Autodesk Fusion 360 part; units mm, degrees
(part 2 of 3)
sketch "Schizzo2" plane through (0, 0, 0) normal (0, -1, 0) x (1, 0, 0)
  line L0 (-21, 0) -> (-5, 0)
  line L1 (-5, 0) -> (-5, 20)
  line L2 (-5, 20) -> (-21, 20)
  line L3 (-21, 20) -> (-21, 0)
  line L4 (-21, 10) -> (-5, 10) construction
  line L5 (-13, 20) -> (-13, 0) construction
  line L6 (-5, 8.5) -> (-21, 8.5)
  line L7 (-21, 8.5) -> (-21, 11.5)
  line L8 (-21, 11.5) -> (-5, 11.5)
  line L9 (-5, 11.5) -> (-5, 8.5)
  line L10 (-5, 8.5) -> (-21, 11.5) construction
  line L11 (-21, 8.5) -> (-5, 11.5) construction
  line L12 (-21, 20) -> (-18, 20) construction
  line L13 (-18, 20) -> (-18, 17) construction
  line L14 (-18, 17) -> (-21, 17) construction
  line L15 (-21, 17) -> (-21, 20) construction
  line L16 (-20, 15) -> (-16, 15)
  line L17 (-16, 15) -> (-16, 19)
  line L18 (-16, 19) -> (-20, 19)
  line L19 (-20, 19) -> (-20, 15)
  line L20 (-20, 15) -> (-16, 19) construction
  line L21 (-16, 15) -> (-20, 19) construction
  point P0 (-13, 10)
  point P1 (-18, 17)
  dimension "d7" = 3
  dimension "d83" = 3
  dimension "d84" = 3
  dimension "d93" = 4
  dimension "d94" = 4
  constraint midpoint L3 L4.start
  constraint midpoint L1 L4.end
  constraint midpoint L2 L5.start
  constraint midpoint L0 L5.end
  constraint horizontal L6
  constraint perpendicular L6 L7
  constraint parallel L6 L8
  constraint parallel L7 L9
  constraint coincident L10 P0
  constraint coincident L11 P0
  constraint coincident L1 L6.start
  constraint midpoint L5 P0
  constraint horizontal L12
  constraint vertical L13
  constraint horizontal L14
  constraint vertical L15
  constraint coincident L2.end L3.start
  constraint horizontal L16
  constraint perpendicular L16 L17
  constraint parallel L16 L18
  constraint parallel L17 L19
  constraint coincident L20 P1
  constraint coincident L21 P1
  constraint coincident P1 L13.end
  measures "d7" distance of L6 L8
  measures "d83" distance of L2.end L12.end
  measures "d84" distance of L2.end L14.end
  measures "d93" distance of L17.end L18.end
  measures "d94" distance of L16.end L17.end
sketch "Schizzo3" plane through (0, 140, 0) normal (0, 1, 0) x (-1, 0, 0)
  line L0 (5, 0) -> (21, 0)
  line L1 (21, 0) -> (21, 20)
  line L2 (21, 20) -> (5, 20)
  line L3 (5, 20) -> (5, 0)
  line L4 (13, 20) -> (13, 1) construction
  line L5 (5, 10) -> (21, 10) construction
  line L6 (21, 8.5) -> (5, 8.5)
  line L7 (5, 8.5) -> (5, 11.5)
  line L8 (5, 11.5) -> (21, 11.5)
  line L9 (21, 11.5) -> (21, 8.5)
  line L10 (21, 8.5) -> (5, 11.5) construction
  line L11 (5, 8.5) -> (21, 11.5) construction
  line L12 (5, 0) -> (8, 0) construction
  line L13 (8, 0) -> (8, 3) construction
  line L14 (8, 3) -> (5, 3) construction
  line L15 (5, 3) -> (5, 0) construction
  line L16 (10, 1) -> (6, 1)
  line L17 (6, 1) -> (6, 5)
  line L18 (6, 5) -> (10, 5)
  line L19 (10, 5) -> (10, 1)
  line L20 (10, 1) -> (6, 5) construction
  line L21 (6, 1) -> (10, 5) construction
  point P0 (13, 10)
  point P1 (8, 3)
  point P2 (17, 16)
  dimension "d8" = 3
  dimension "d87" = 3
  dimension "d88" = 3
  dimension "d89" = 4
  dimension "d90" = 4
  constraint midpoint L2 L4.start
  constraint perpendicular L0 L4
  constraint midpoint L3 L5.start
  constraint midpoint L1 L5.end
  constraint horizontal L6
  constraint perpendicular L6 L7
  constraint parallel L6 L8
  constraint parallel L7 L9
  constraint coincident L10 P0
  constraint coincident L11 P0
  constraint coincident L1 L6.start
  constraint midpoint L5 P0
  constraint horizontal L12
  constraint vertical L13
  constraint horizontal L14
  constraint vertical L15
  constraint coincident L0.start L3.end
  constraint horizontal L16
  constraint perpendicular L16 L17
  constraint parallel L16 L18
  constraint parallel L17 L19
  constraint coincident L20 P1
  constraint coincident L21 P1
  constraint coincident P1 L13.end
  measures "d8" distance of L6 L8
  measures "d87" distance of L0.start L12.end
  measures "d88" distance of L0.start L14.end
  measures "d89" distance of L17.end L18.end
  measures "d90" distance of L16.end L17.end
extrude "Estrusione28" cut sketch "Schizzo2" against normal blind 1 contours L16 L17 L18 L19 bodies 1
extrude "Estrusione29" cut sketch "Schizzo3" against normal blind 1 contours L16 L17 L18 L19 bodies 1
ref_plane "Piano di lavoro2" through (-8, 140, 0) normal (-0.997459, 0.071247, 0) x (-0.071247, -0.997459, 0)
sketch "Schizzo8" plane through (-17.9086, 1.2792, 0) normal (-0.997459, 0.071247, 0) x (-0.071247, -0.997459, 0)
  line L0 (1, 16) -> (-139.3, 4)
pipe "Tubo1" cut square section size 4 path "Schizzo8" along L0 bodies 1
sketch "Schizzo11" plane through (-5, 0, 0) normal (1, 0, 0) x (0, 1, 0)
  line L0 (0, 0) -> (140, 0)
  line L1 (140, 0) -> (140, 20)
  line L2 (140, 20) -> (0, 20)
  line L3 (0, 20) -> (0, 0)
  line L4 (140, 3) -> (123.5, 3) construction
  line L5 (131.75, 3) -> (131.75, 0) construction
  line L6 (123.5, 5) -> (140, 5)
  line L7 (140, 5) -> (140, 1)
  line L8 (140, 1) -> (123.5, 1)
  line L9 (123.5, 1) -> (123.5, 5)
  line L10 (123.5, 5) -> (140, 1) construction
  line L11 (140, 5) -> (123.5, 1) construction
  line L12 (0, 0) -> (140, 0)
  point P0 (131.75, 3)
  point P1 (140, 3)
  dimension "d129" = 16.5
  dimension "d132" = 4
  constraint coincident L1 P1
  constraint perpendicular L1 L4
  constraint midpoint L4 P0
  constraint coincident L0 L5.end
  constraint perpendicular L0 L5
  constraint horizontal L6
  constraint perpendicular L6 L7
  constraint parallel L6 L8
  constraint parallel L7 L9
  constraint coincident L10 P0
  constraint coincident L11 P0
  constraint coincident P0 L5.start
  constraint coincident P1 L7
  constraint coincident P1 L4.start
  measures "d129" distance of P1 L4.end
  measures "d132" distance of L6 L8
extrude "Estrusione37" cut sketch "Schizzo11" against normal blind 5 contours L1 L6 L7 L8 L9 bodies 1
sketch "Schizzo12" plane through (-21, 0, 0) normal (-1, 0, 0) x (0, -1, 0)
  line L0 (-140, 0) -> (0, 0)
  line L1 (0, 0) -> (0, 20)
  line L2 (0, 20) -> (-140, 20)
  line L3 (-140, 20) -> (-140, 0)
  line L4 (0, 17) -> (-16.5, 17) construction
  line L5 (-8.25, 17) -> (-8.25, 20) construction
  line L6 (0, 15) -> (-16.5, 15)
  line L7 (-16.5, 15) -> (-16.5, 19)
  line L8 (-16.5, 19) -> (0, 19)
  line L9 (0, 19) -> (0, 15)
  line L10 (0, 15) -> (-16.5, 19) construction
  line L11 (-16.5, 15) -> (0, 19) construction
  point P0 (0, 17)
  point P1 (-8.25, 17)
  dimension "d135" = 16.5
  dimension "d136" = 4
  constraint coincident L1 P0
  constraint perpendicular L1 L4
  constraint coincident P0 L4.start
  constraint midpoint L4 P1
  constraint coincident L2 L5.end
  constraint perpendicular L2 L5
  constraint horizontal L6
  constraint perpendicular L6 L7
  constraint parallel L6 L8
  constraint parallel L7 L9
  constraint coincident L10 P1
  constraint coincident L11 P1
  constraint coincident P1 L5.start
  constraint collinear L1 L9
  measures "d135" distance of P0 L4.end
  measures "d136" distance of L6 L8
extrude "Estrusione38" cut sketch "Schizzo12" against normal blind 5 contours L1 L6 L7 L8 L9 bodies 1
extrude "Estrusione2" cut sketch "Schizzo3" against normal blind 16.5 contours L1 L3 L6 L7 L8 L9 bodies 1
extrude "Estrusione3" cut sketch "Schizzo2" against normal blind 16.5 contours L1 L3 L6 L7 L8 L9 bodies 1
extrude "Estrusione4" cut sketch "Schizzo1" along normal blind 20 contours L0 L3 A0 L118 | L0 L1 A0 L118 | L3 A0 L118 L119 | L1 A0 L117 L118 | L3 A2 L122 L123 | L1 A2 L122 L125 | L2 L3 A2 L122 | L1 L2 A2 L122 bodies 1
extrude "Estrusione26" cut sketch "Schizzo1" along normal blind 1 contours L4 A1 A11 | L4 A1 A11 | L4 A3 A12 | L4 A3 A12 bodies 1
extrude "Estrusione120" cut sketch "Schizzo1" along normal blind 0.5 contours A0 A1 L116 L118 | L3 A0 L116 L119 picked at (-19.6721, 8.4598) bodies 1
sketch "Schizzo6" plane through (0, 0, 20) normal (0, 0, 1) x (-1, 0, 0)
  arc A0 (21, -8) -> (5, -8) centre (13, -8) ccw
  line L0 (5, -8) -> (5, -132)
  arc A1 (5, -132) -> (21, -132) centre (13, -132) ccw
  line L1 (21, -132) -> (21, -8)
  circle A2 centre (13, -132) radius 2
  circle A3 centre (13, -8) radius 2
  line L2 (13, -132) -> (13, -8) construction
  circle A4 centre (13, -132) radius 4
  line L3 (21, -70) -> (5, -70) construction
  circle A5 centre (13, -8) radius 4
  line L4 (5, -128) -> (21, -128)
  line L5 (21, -128) -> (21, -136)
  line L6 (21, -136) -> (5, -136)
  line L7 (5, -136) -> (5, -128)
  line L8 (5, -128) -> (21, -136) construction
  line L9 (21, -128) -> (5, -136) construction
  point P0 (13, -132)
  dimension "d78" = 8
  constraint coincident P0 A1.centre
  constraint coincident A0.centre A3.centre
  constraint midpoint L1 L3.start
  constraint midpoint L0 L3.end
  constraint symmetric A4 L3 A5
  constraint horizontal L4
  constraint perpendicular L4 L5
  constraint parallel L4 L6
  constraint parallel L5 L7
  constraint coincident L8 P0
  constraint coincident L9 P0
  constraint tangent A4 L6
  constraint collinear L1 L5
  measures "d78" diameter of A4
extrude "Estrusione27" cut sketch "Schizzo6" against normal blind 1 contours A4 | A5 bodies 1
extrude "Estrusione121" cut sketch "Schizzo6" against normal blind 0.5 contours L0 A1 A4 L4 L6 L7 bodies 1
extrude "Estrusione19" add sketch "Schizzo1" along normal blind 28 separate body contours L7 L11 A5 | L7 L11 A7 makes body 2
extrude "Estrusione18" add sketch "Schizzo1" along normal blind 4 contours L10 A4 A8 | L10 A4 A8 | L9 L10 L11 A4 | L10 A8 L16 | L10 A8 L16 | L7 L10 A4 A5 | L9 L10 L11 A6 | L10 L13 L14 L15 L16 A9 | L10 L12 L13 L16 L17 A9 | A8 L15 | A8 L17 | L7 L11 A5 | L10 A6 L18 L19 L22 L23 | L7 L11 A7 | L7 L10 A6 A7 | L10 A8 L13 | L10 A8 L13 | L10 A9 | L10 A9 | A8 L14 | A8 L12 | L10 A6 L19 L20 L21 L22 | L10 L19 L20 L21 L22 A10 | L10 L18 L19 L22 L23 A10 | L10 A10 | L10 A10 bodies 2
extrude "Estrusione20" cut sketch "Schizzo1" along normal blind 4 contours L10 A9 | L10 A9 | L10 A10 | L10 A10 bodies 2
extrude "Estrusione21" cut sketch "Schizzo1" along normal blind 2 contours L10 L13 L14 L15 L16 A9 | L10 L12 L13 L16 L17 A9 | L10 L19 L20 L21 L22 A10 | L10 L18 L19 L22 L23 A10 bodies 2
extrude "Estrusione22" add 1 faces at (28.834, 17.1558, 4) along direction (0, 0, 1) blind 3 from surface at 8.5 on bodies 2 bodies 2
extrude "Estrusione23" add 1 faces at (28.834, 17.1558, 15.5) along direction (0, 0, 1) blind 4 from surface at 8.5 on bodies 2 bodies 2
sketch "Schizzo5" plane through (0, 0, 28) normal (0, 0, 1) x (-1, 0, 0)
  circle A0 centre (-34.1674, -25.6558) radius 1.6
  circle A1 centre (-34.1674, -8.6558) radius 1.6
  line L0 (-42.1674, -8.6558) -> (-42.1674, -25.6558)
  arc A2 (-42.1674, -25.6558) -> (-26.1674, -25.6558) centre (-34.1674, -25.6558) ccw
  line L1 (-26.1674, -25.6558) -> (-26.1674, -8.6558)
  arc A3 (-26.1674, -8.6558) -> (-42.1674, -8.6558) centre (-34.1674, -8.6558) ccw
  line L2 (-34.1674, -8.6558) -> (-34.1674, -25.6558) construction
  circle A4 centre (-34.1674, -8.6558) radius 3
  circle A5 centre (-34.1674, -25.6558) radius 3
  circle A6 centre (-34.1674, -8.6558) radius 4
  circle A7 centre (-34.1674, -25.6558) radius 4
  dimension "d67" = 6
  dimension "d68" = 6
  dimension "d69" = 8
  dimension "d70" = 8
  constraint coincident A1.centre A3.centre
  constraint coincident A0.centre A2.centre
  constraint concentric A4 A6
  measures "d67" diameter of A4
  measures "d68" diameter of A5
  measures "d69" diameter of A6
  measures "d70" diameter of A7
extrude "Estrusione25" add sketch "Schizzo5" against normal blind 5 contours A4 | A5 | A6 | A7 bodies 2
extrude "Estrusione24" cut sketch "Schizzo5" against normal blind 3.2 contours A4 | A5 bodies 2
extrude "Estrusione97" add sketch "Schizzo1" along normal blind 8 separate body contours L172 L174 L175 L176 L183 | L174 L175 L176 L178 L374 L375 | L172 L173 L175 L176 L190 | L174 L178 L179 L278 L290 | L174 L178 L278 L281 L290 L375 | L173 L175 L176 L178 L373 L374 | L175 L178 L180 L278 L372 L375 | L175 L178 L374 L375 | L175 L178 L373 L374 | L175 L178 L180 L278 L372 L373 | L173 L178 L274 L278 L283 L373 | L173 L177 L178 L278 L283 makes body 3
extrude "Estrusione98" add sketch "Schizzo1" along normal blind 28.5 from surface at 8 contours L174 L178 L179 L278 L290 | L174 L178 L278 L281 L290 L375 | L175 L178 L180 L278 L372 L375 | L175 L178 L180 L278 L372 L373 | L173 L178 L274 L278 L283 L373 | L173 L177 L178 L278 L283 bodies 3
extrude "Estrusione138" cut sketch "Schizzo1" along normal blind 3 contours L175 L178 L180 L278 L372 L375 | L175 L178 L374 L375 | L175 L178 L373 L374 | L175 L178 L180 L278 L372 L373 bodies 3
extrude "Estrusione102" add sketch "Schizzo1" along normal blind 11 contours L172 L183 L184 L185 L186 | L172 L187 L188 L189 L190 bodies 3
extrude "Estrusione99" add sketch "Schizzo1" along normal blind 2.8 contours L278 L279 L281 L282 L287 L288 L290 | L278 L280 L281 L282 L288 | L274 L275 L276 L278 L284 | L274 L276 L277 L278 L283 L284 L285 bodies 3
extrude "Estrusione101" add sketch "Schizzo1" along normal blind 4 from surface at 8 contours L278 L279 L287 L289 L290 | L278 L279 L281 L282 L287 L288 L290 | L277 L278 L283 L285 L286 | L274 L276 L277 L278 L283 L284 L285 bodies 3
sketch "Schizzo45" plane through (0, 44.5, 0) normal (0, 1, 0) x (-1, 0, 0)
  line L0 (335.0462, 12) -> (341.0462, 12)
  line L1 (341.0462, 12) -> (341.0462, 36.5)
  line L2 (308.0462, 36.5) -> (308.0462, 12)
  line L3 (308.0462, 12) -> (314.0462, 12)
  line L4 (314.0462, 12) -> (314.0462, 8)
  line L5 (314.0462, 8) -> (308.0462, 8)
  line L6 (308.0462, 8) -> (308.0462, 0)
  line L7 (308.0462, 0) -> (312.1462, 0)
  line L8 (312.1462, 0) -> (312.1462, 2.8)
  line L9 (312.1462, 2.8) -> (318.8462, 2.8)
  line L10 (318.8462, 2.8) -> (318.8462, 3)
  line L11 (330.2462, 2.8) -> (336.9462, 2.8)
  line L12 (336.9462, 2.8) -> (336.9462, 0)
  line L13 (336.9462, 0) -> (341.0462, 0)
  line L14 (341.0462, 0) -> (341.0462, 8)
  line L15 (341.0462, 8) -> (335.0462, 8)
  line L16 (335.0462, 8) -> (335.0462, 12)
  line L17 (308.0462, 40) -> (341.0462, 40) construction
  line L18 (341.0462, 40) -> (341.0462, 0) construction
  line L19 (341.0462, 0) -> (308.0462, 0) construction
  line L20 (308.0462, 0) -> (308.0462, 40) construction
  line L21 (308.0462, 20) -> (341.0462, 20) construction
  circle A0 centre (324.5462, 22.25) radius 14.25
  line L22 (308.0462, 28.25) -> (341.0462, 28.25)
  line L23 (308.0462, 0) -> (341.0462, 0)
  line L24 (324.5462, 0) -> (324.5462, 36.5) construction
  line L25 (318.8462, 3) -> (330.2462, 3)
  line L26 (330.2462, 3) -> (330.2462, 2.8)
  line L27 (341.0462, 36.5) -> (308.0462, 36.5)
  dimension "d560" = 28.5
  dimension "d561" = 6
  dimension "d584" = 22.25
  constraint horizontal L17
  constraint vertical L18
  constraint horizontal L19
  constraint vertical L20
  constraint coincident L13.end L14.start
  constraint midpoint L20 L21.start
  constraint midpoint L18 L21.end
  constraint coincident L2 L22.start
  constraint coincident L18 L22.end
  constraint perpendicular L18 L22
  constraint midpoint L23 L24.start
  constraint coincident A0.centre L24
  measures "d560" diameter of A0
  measures "d561" distance of A0.centre L22
  measures "d584" distance of A0.centre L23
extrude "Estrusione128" cut sketch "Schizzo45" against normal blind 7 contours A0 L22 | A0 L22 bodies 3
extrude "Estrusione139" cut sketch "Schizzo45" against normal blind 5 contours L1 A0 L22 L27 | L2 A0 L22 L27 bodies 3
extrude "Estrusione84" add sketch "Schizzo1" along normal blind 1 separate body contours L129 L131 L133 L135 L147 L148 | L131 L133 L141 L148 | L129 L131 L133 L135 L146 L147 | L130 L131 L141 L148 | L131 L133 L141 L146 | L130 L131 L143 L148 | L130 L131 L141 L146 | L131 L139 L143 L148 | L130 L131 L143 L146 | L127 L131 L138 L139 L148 L149 | L131 L139 L143 L146 | L127 L131 L138 L139 L146 L149 makes body 4
extrude "Estrusione85" add sketch "Schizzo1" along normal blind 16 contours L126 L129 L132 L133 L135 L148 | L129 L131 L133 L135 L147 L148 | L126 L130 L141 L142 L148 | L129 L131 L133 L135 L146 L147 | L126 L130 L142 L143 L148 | L130 L131 L141 L148 | L128 L129 L133 L134 L135 L146 | L130 L131 L143 L148 | L130 L131 L141 L146 | L126 L127 L136 L138 L139 L148 | L130 L131 L143 L146 | L128 L130 L140 L141 L146 | L127 L131 L138 L139 L148 L149 | L128 L130 L140 L143 L146 | L127 L131 L138 L139 L146 L149 | L127 L128 L137 L138 L139 L146 bodies 4
sketch "Schizzo32" plane through (88, 0, 0) normal (1, 0, 0) x (0, 1, 0)
  line L0 (-8, 0) -> (30, 0)
  line L1 (30, 0) -> (30, 16)
  line L2 (30, 16) -> (-8, 16)
  line L3 (-8, 16) -> (-8, 0)
  line L4 (-8, 16) -> (30, 16) construction
  line L5 (30, 16) -> (30, 0) construction
  line L6 (30, 0) -> (-8, 0) construction
  line L7 (-8, 0) -> (-8, 16) construction
  line L8 (-8, 8) -> (30, 8) construction
  line L9 (11, 16) -> (11, 0) construction
  circle A0 centre (0, 8) radius 8
  circle A1 centre (22, 8) radius 8
  circle A2 centre (0, 8) radius 1.6
  circle A3 centre (0, 8) radius 3.25
  circle A4 centre (22, 8) radius 3.25
  circle A5 centre (22, 8) radius 1.6
  line L10 (-8, 4) -> (30, 4) construction
  line L11 (6.9282, 4) -> (15.0718, 4) construction
  line L12 (6.9282, 4) -> (15.0718, 4)
  line L13 (0.0738, 11.2492) -> (-2.777, 9.6885)
  line L14 (-2.777, 9.6885) -> (-2.8508, 6.4393)
  line L15 (-2.8508, 6.4393) -> (-0.0738, 4.7508)
  line L16 (-0.0738, 4.7508) -> (2.777, 6.3115)
  line L17 (2.777, 6.3115) -> (2.8508, 9.5607)
  line L18 (2.8508, 9.5607) -> (0.0738, 11.2492)
  line L19 (21.9262, 11.2492) -> (24.777, 9.6885)
  line L20 (19.1492, 9.5607) -> (21.9262, 11.2492)
  line L21 (19.223, 6.3115) -> (19.1492, 9.5607)
  line L22 (22.0738, 4.7508) -> (19.223, 6.3115)
  line L23 (24.8508, 6.4393) -> (22.0738, 4.7508)
  line L24 (24.777, 9.6885) -> (24.8508, 6.4393)
  circle A6 centre (0, 8) radius 4
  circle A7 centre (22, 8) radius 4
  point P0 (0, 8)
  dimension "d369" = 22
  dimension "d370" = 3.2
  dimension "d371" = 6.5
  dimension "d372" = 4
  dimension "d380" = 8
  constraint horizontal L4
  constraint vertical L5
  constraint horizontal L6
  constraint vertical L7
  constraint coincident L2.end L3.start
  constraint coincident L0.end L1.start
  constraint midpoint L7 L8.start
  constraint midpoint L5 L8.end
  constraint midpoint L4 L9.start
  constraint midpoint L6 L9.end
  constraint coincident L8 P0
  constraint tangent L4 A0
  constraint tangent L7 A0
  constraint symmetric L9 A0 A1
  constraint concentric A0 A2
  constraint concentric A0 A3
  constraint symmetric L9 A2 A5
  constraint symmetric L9 A3 A4
  constraint coincident L7 L10.start
  constraint coincident L5 L10.end
  constraint perpendicular L5 L10
  constraint coincident L10 L11.start
  constraint coincident A0 L11.start
  constraint coincident A1 L11.end
  constraint coincident L10 L11.end
  constraint coincident A3 L13.start
  constraint coincident P0 A0.centre
  constraint symmetric L9 L13.start L19.start
  constraint symmetric L9 L13.end L19.end
  constraint symmetric L9 L14.end L23.start
  constraint symmetric L9 L15.end L22.start
  constraint symmetric L9 L16.end L21.start
  constraint symmetric L9 L17.end L20.start
  constraint concentric A3 A6
  constraint symmetric L9 A6 A7
  measures "d369" distance of P0 A1.centre
  measures "d370" diameter of A2
  measures "d371" diameter of A3
  measures "d372" distance of L6 L10
  measures "d380" diameter of A6
extrude "Estrusione86" cut sketch "Schizzo32" against normal blind 28 contours L0 L3 A0 | L2 L3 A0 | L0 L1 A1 | L1 L2 A1 | A2 | A5 bodies 4
extrude "Estrusione87" add sketch "Schizzo32" against normal blind 28 contours L0 A0 A1 L12 bodies 4
extrude "Estrusione89" add sketch "Schizzo32" along normal blind 5 from surface at -28 contours A3 L17 | A3 L18 | L13 L14 L15 L16 L17 L18 | A3 L16 | A3 L13 | A3 L15 | A3 L14 | A4 L24 | A4 L19 | L19 L20 L21 L22 L23 L24 | A4 L23 | A4 L20 | A4 L22 | A4 L21 | A6 | A7 bodies 4
extrude "Estrusione91" cut sketch "Schizzo32" against normal blind 2 contours L13 L14 L15 L16 L17 L18 | L19 L20 L21 L22 L23 L24 bodies 4
extrude "Estrusione88" cut sketch "Schizzo32" along normal blind 3.2 from surface at -28 contours A3 L17 | A3 L18 | L13 L14 L15 L16 L17 L18 | A3 L16 | A3 L13 | A3 L15 | A3 L14 | A4 L24 | A4 L19 | L19 L20 L21 L22 L23 L24 | A4 L23 | A4 L20 | A4 L22 | A4 L21 bodies 4
sketch "Schizzo40" plane through (-310.0462, 0, 0) normal (1, 0, 0) x (0, 1, 0)
  line L0 (-8, 0) -> (39.5, 0)
  line L1 (39.5, 8) -> (-2, 8)
  line L2 (-2, 8) -> (-2, 11)
  line L3 (-2, 11) -> (-8, 11)
  line L4 (-8, 11) -> (-8, 0)
  line L5 (-8, 11) -> (39.5, 11) construction
  line L6 (39.5, 11) -> (39.5, 0) construction
  line L7 (39.5, 0) -> (-8, 0) construction
  line L8 (-8, 0) -> (-8, 11) construction
  line L9 (-2, 8) -> (-8, 8) construction
  line L10 (-2, 11) -> (-3, 8)
  line L11 (-3, 8) -> (-2, 8)
  line L12 (39.5, 11) -> (44.5, 11) construction
  line L13 (44.5, 11) -> (44.5, 0) construction
  line L14 (44.5, 0) -> (39.5, 0) construction
  line L15 (39.5, 0) -> (39.5, 11) construction
  line L16 (44.5, 0) -> (47, 0) construction
  line L17 (47, 0) -> (47, 11) construction
  line L18 (47, 11) -> (44.5, 11) construction
  line L19 (44.5, 11) -> (44.5, 0) construction
  line L20 (44.5, 8) -> (47, 8) construction
  line L21 (44.5, 3) -> (47, 3) construction
  line L22 (44.5, 9) -> (47, 9) construction
  line L23 (44.5, 2) -> (47, 2) construction
  line L24 (44.5, 9) -> (47, 8)
  line L25 (44.5, 8) -> (47, 8)
  line L26 (44.5, 8) -> (44.5, 9)
  line L27 (47, 3) -> (44.5, 3)
  line L28 (44.5, 3) -> (44.5, 2)
  line L29 (44.5, 2) -> (47, 3)
  line L30 (39.5, 0) -> (39.5, 8)
  dimension "d447" = 1
  dimension "d450" = 5
  dimension "d451" = 2.5
  dimension "d453" = 3
  dimension "d454" = 3
  dimension "d455" = 1
  dimension "d456" = 1
  constraint horizontal L5
  constraint vertical L6
  constraint horizontal L7
  constraint vertical L8
  constraint coincident L0.end L6.end
  constraint coincident L3.end L4.start
  constraint coincident L1.end L2.start
  constraint coincident L8 L9.end
  constraint perpendicular L8 L9
  constraint coincident L2.end L3.start
  constraint coincident L9 L10.end
  constraint horizontal L12
  constraint vertical L13
  constraint horizontal L14
  constraint vertical L15
  constraint horizontal L16
  constraint vertical L17
  constraint horizontal L18
  constraint vertical L19
  constraint collinear L12 L18
  constraint collinear L7 L16
  constraint coincident L19 L20.start
  constraint coincident L17 L20.end
  constraint perpendicular L17 L20
  constraint coincident L13 L21.start
  constraint coincident L17 L21.end
  constraint coincident L13 L22.start
  constraint coincident L17 L22.end
  constraint perpendicular L17 L22
  constraint coincident L19 L23.start
  constraint coincident L17 L23.end
  measures "d447" distance of L2 L10.end
  measures "d450" distance of L5.end L12.end
  measures "d451" distance of L13.end L16.end
  measures "d453" distance of L17.end L20.end
  measures "d454" distance of L16 L21
  measures "d455" distance of L20 L22
  measures "d456" distance of L21 L23
extrude "Estrusione103" cut sketch "Schizzo40" against normal blind 30 contours L2 L10 L11 bodies 3
extrude "Estrusione104" cut sketch "Schizzo40" along normal mid plane 60 contours L24 L25 L26 | L27 L28 L29 bodies 3
extrude "Estrusione39" add sketch "Schizzo1" along normal blind 3 from surface at 15 separate body contours L24 L27 L29 L31 L32 L33 | L24 L29 L31 L36 A14 | L26 L27 L29 L30 L31 L33 | L24 L28 L35 L36 A14 | L26 L29 L31 L36 A14 | L24 L28 L35 L38 A14 | L29 L36 L41 L42 L47 L48 A13 A14 | L28 L36 A13 A14 | L29 L36 L42 L43 L48 L49 A13 A14 | L24 L29 L34 L38 A14 | L28 L38 A13 A14 | L29 L36 L42 L48 A13 | L28 L29 L36 L41 L47 | L41 L42 L47 L48 A13 | L28 L41 L47 A13 | L29 L42 L48 A13 | L29 L42 L48 A13 | L28 L36 A13 A14 | L26 L28 L36 L37 A14 | L24 L25 L29 L34 | L29 L38 L41 L44 L47 L50 A13 A14 | L28 L41 L47 A13 | L28 L29 L36 L43 L49 | L29 L36 L42 L48 A13 | L28 L29 L38 L41 L47 | L42 L43 L48 L49 A13 | L28 L43 L49 A13 | L28 L38 A13 A14 | L26 L28 L37 L38 A14 | L25 L26 L29 L34 | L26 L29 L34 L38 A14 | L41 L44 L47 L50 A13 | L29 L38 L44 L50 A13 | L29 L38 L43 L44 L49 L50 A13 A14 | L28 L29 L38 L43 L49 | L28 L43 L49 A13 | L29 L38 L44 L50 A13 | L29 L44 L50 A13 | L29 L44 L50 A13 | L43 L44 L49 L50 A13 makes body 5
extrude "Estrusione40" add sketch "Schizzo1" along normal blind 22 from surface at 15 contours L24 L27 L29 L31 L32 L33 | L26 L27 L29 L30 L31 L33 | L24 L28 L35 L36 A14 | L24 L28 L35 L38 A14 | L28 L36 A13 A14 | L28 L38 A13 A14 | L28 L29 L36 L41 L47 | L28 L41 L47 A13 | L28 L36 A13 A14 | L26 L28 L36 L37 A14 | L24 L25 L29 L34 | L28 L41 L47 A13 | L28 L29 L36 L43 L49 | L28 L29 L38 L41 L47 | L28 L43 L49 A13 | L28 L38 A13 A14 | L26 L28 L37 L38 A14 | L25 L26 L29 L34 | L28 L29 L38 L43 L49 | L28 L43 L49 A13 bodies 5
extrude "Estrusione41" cut sketch "Schizzo1" along normal blind 8 from surface at 15 contours L29 L36 L42 L48 A13 | L28 L29 L36 L41 L47 | L41 L42 L47 L48 A13 | L28 L29 L36 L43 L49 | L29 L36 L42 L48 A13 | L28 L29 L38 L41 L47 | L42 L43 L48 L49 A13 | L41 L44 L47 L50 A13 | L29 L38 L44 L50 A13 | L28 L29 L38 L43 L49 | L29 L38 L44 L50 A13 | L43 L44 L49 L50 A13 bodies 5
sketch "Schizzo13" plane through (-130.5, 0, 0) normal (-1, 0, 0) x (0, -1, 0)
  line L0 (-16, 15) -> (0, 15)
  line L1 (0, 15) -> (0, 37)
  line L2 (0, 37) -> (-16, 37)
  line L3 (-16, 37) -> (-16, 15)
  line L4 (-8, 37) -> (-8, 15)
  circle A0 centre (-8, 29) radius 8
  circle A1 centre (-8, 29) radius 1.6
  line L5 (-6.1897, 26.3009) -> (-4.7573, 29.2183)
  line L6 (-4.7573, 29.2183) -> (-6.5677, 31.9174)
  line L7 (-6.5677, 31.9174) -> (-9.8103, 31.6991)
  line L8 (-9.8103, 31.6991) -> (-11.2427, 28.7817)
  line L9 (-11.2427, 28.7817) -> (-9.4323, 26.0826)
  line L10 (-9.4323, 26.0826) -> (-6.1897, 26.3009)
  point P0 (-8, 29)
  dimension "d153" = 16
  dimension "d154" = 3.2
  dimension "d157" = 3.25
  constraint midpoint L2 L4.start
  constraint midpoint L0 L4.end
  constraint tangent L3 A0
  constraint tangent L2 A0
  constraint tangent L1 A0
  constraint concentric A0 A1
  constraint coincident P0 A0.centre
  measures "d153" diameter of A0
  measures "d154" diameter of A1
  measures "d157" distance of L5.start P0
sketch "Schizzo14" plane through (-102.5, 0, 0) normal (1, 0, 0) x (0, 1, 0)
  line L0 (0, 15) -> (16, 15)
  line L1 (16, 15) -> (16, 37)
  line L2 (16, 37) -> (0, 37)
  line L3 (0, 37) -> (0, 15)
  line L4 (8, 37) -> (8, 15)
  circle A0 centre (8, 29) radius 8 construction
  circle A1 centre (8, 29) radius 3
  circle A2 centre (8, 29) radius 4
  dimension "d160" = 6
  dimension "d163" = 8
  constraint midpoint L2 L4.start
  constraint midpoint L0 L4.end
  constraint tangent L3 A0
  constraint tangent L2 A0
  constraint tangent L1 A0
  constraint concentric A0 A1
  constraint concentric A1 A2
  measures "d160" diameter of A1
  measures "d163" diameter of A2
extrude "Estrusione43" cut sketch "Schizzo13" against normal blind 2 contours L4 A1 L7 L8 L9 L10 | L4 A1 L5 L6 L7 L10 bodies 5
extrude "Estrusione45" add sketch "Schizzo14" against normal blind 5 contours L4 A1 A2 | L4 A1 A2 | L4 A1 | L4 A1 bodies 5
extrude "Estrusione44" cut sketch "Schizzo14" against normal blind 3.2 contours L4 A1 | L4 A1 bodies 5
extrude "Estrusione42" cut sketch "Schizzo13" against normal blind 28 contours L2 L3 A0 | L1 L2 A0 | L4 A1 | L4 A1 bodies 5
extrude "Estrusione46" add sketch "Schizzo1" along normal blind 18 contours L29 L36 L41 L42 L47 L48 A13 A14 | L28 L36 A13 A14 | L29 L36 L42 L43 L48 L49 A13 A14 | L28 L38 A13 A14 | L41 L42 L47 L48 A13 | L28 L36 A13 A14 | L29 L38 L41 L44 L47 L50 A13 A14 | L42 L43 L48 L49 A13 | L28 L38 A13 A14 | L41 L44 L47 L50 A13 | L29 L38 L43 L44 L49 L50 A13 A14 | L43 L44 L49 L50 A13 bodies 5
ref_plane "Piano di lavoro3" through (-116.5, 8, 26) normal (0, -1, 0) x (1, 0, 0)
sketch "Schizzo15" plane through (0, 8, 0) normal (0, -1, 0) x (-1, 0, 0)
  line L0 (130.5, -15) -> (102.5, -15) construction
  line L1 (102.5, -15) -> (102.5, -8.9) construction
  line L2 (102.5, -8.9) -> (130.5, -8.9) construction
  line L3 (130.5, -8.9) -> (130.5, -15) construction
  line L4 (130.5, 0) -> (102.5, 0) construction
  line L5 (130.5, -8.9) -> (102.5, -8.9) construction
  line L6 (102.5, -8.9) -> (102.5, -2.8) construction
  line L7 (102.5, -2.8) -> (130.5, -2.8) construction
  line L8 (130.5, -2.8) -> (130.5, -8.9) construction
  line L9 (116.5, -2.8) -> (116.5, -15) construction
  line L10 (121.5, -8.9) -> (120.5, -8.9)
  line L11 (120.5, -8.9) -> (120.5, -13.1)
  line L12 (120.5, -13.1) -> (121.5, -13.1)
  line L13 (121.5, -13.1) -> (121.5, -8.9)
  line L14 (121.5, -15) -> (121.5, -2.8) construction
  line L15 (121.5, -7) -> (120.5, -7)
  line L16 (120.5, -7) -> (120.5, -2.8)
  line L17 (120.5, -2.8) -> (121.5, -2.8)
  line L18 (121.5, -2.8) -> (121.5, -7)
  point P0 (130.5, 0)
  point P1 (102.5, 0)
  point P2 (130.5, -15)
  point P3 (102.5, -15)
  dimension "d169" = 6.1
  dimension "d170" = 6.1
  dimension "d171" = 1
  dimension "d172" = 4.2
  dimension "d173" = 5
  dimension "d174" = 1
  dimension "d175" = 4.2
  constraint horizontal L0
  constraint vertical L1
  constraint horizontal L2
  constraint vertical L3
  constraint horizontal L5
  constraint vertical L6
  constraint horizontal L7
  constraint vertical L8
  constraint coincident L2.end L3.start
  constraint coincident L1.end L2.start
  constraint midpoint L7 L9.start
  constraint midpoint L0 L9.end
  constraint horizontal L10
  constraint vertical L11
  constraint horizontal L12
  constraint vertical L13
  constraint coincident L2 L10.start
  constraint coincident L0 L14.start
  constraint coincident L7 L14.end
  constraint perpendicular L7 L14
  constraint collinear L13 L14
  constraint horizontal L15
  constraint vertical L16
  constraint horizontal L17
  constraint vertical L18
  constraint coincident L14.end L17.end
  constraint coincident P2 L0.start
  constraint coincident P3 L0.end
  measures "d169" distance of P2 L2.end
  measures "d170" distance of L2.end L7.end
  measures "d171" distance of L10.start L10.end
  measures "d172" distance of L10.start L12.end
  measures "d173" distance of L9 L14
  measures "d174" distance of L15.start L15.end
  measures "d175" distance of L15.start L14.end
revolve "Rivoluzione1" cut sketch "Schizzo15" angle 360 about axis through (-116.5, 8, 2.8) along (0, 0, 1) bodies 5
extrude "Estrusione48" add sketch "Schizzo1" along normal blind 2 separate body contours L53 L56 L59 L60 L61 L64 | L53 L54 L59 L64 | L55 L56 L58 L59 L61 L62 L64 L65 | L54 L55 L59 L62 L63 L64 makes body 6
extrude "Estrusione49" add sketch "Schizzo1" along normal blind 29 contours L53 L56 L59 L60 L61 L64 | L55 L56 L58 L59 L61 L62 L64 L65 bodies 6
extrude "Estrusione52" add sketch "Schizzo1" along normal blind 2 from surface at 27 contours L53 L54 L59 L64 | A15 bodies 6
extrude "Estrusione50" add sketch "Schizzo1" along normal blind 29 contours L54 L55 L59 L62 L63 L64 bodies 6
sketch "Schizzo18" plane through (-135.9612, 0, 0) normal (-1, 0, 0) x (0, -1, 0)
  line L0 (-79.7916, 0) -> (-39.7916, 0)
  line L1 (-39.7916, 0) -> (-39.7916, 29)
  line L2 (-39.7916, 29) -> (-79.7916, 29)
  line L3 (-79.7916, 29) -> (-79.7916, 0)
  line L4 (-65.7416, 0) -> (-65.7416, 29) construction
  line L5 (-56.7416, 0) -> (-56.7416, 29) construction
  line L6 (-39.7916, 0) -> (-79.7916, 0) construction
  line L7 (-39.7916, 12) -> (-79.7916, 12) construction
  circle A0 centre (-56.7416, 12) radius 2.95
  circle A1 centre (-74.7416, 12) radius 2.95
  line L8 (-39.7916, 0) -> (-79.7916, 0)
  point P0 (-65.7416, 0)
  dimension "d224" = 9
  dimension "d225" = 5.9
  dimension "d247" = 12
  dimension "d609" = 14.05
  constraint coincident L2 L4.end
  constraint perpendicular L2 L4
  constraint coincident P0 L4.start
  constraint coincident L0 L5.start
  constraint coincident L2 L5.end
  constraint perpendicular L2 L5
  constraint coincident L0.end L1.start
  constraint coincident L0.start L3.end
  constraint coincident L1 L7.start
  constraint coincident L3 L7.end
  constraint perpendicular L3 L7
  constraint coincident L7 A0.centre
  constraint coincident L5 A0.centre
  constraint symmetric L4 A0 A1
  measures "d224" distance of L4 L5
  measures "d225" diameter of A0
  measures "d247" distance of L7 L8
  measures "d609" distance of L3 L4
extrude "Estrusione57" cut sketch "Schizzo18" against normal blind 2 contours A0 | A1 bodies 6
extrude "Estrusione62" add sketch "Schizzo1" along normal blind 5.5 separate body contours L68 L69 L70 L71 L75 L77 L78 L82 L83 L84 | L71 L75 L76 L77 L78 | L69 L81 L82 L83 L84 makes body 7
extrude "Estrusione63" cut sketch "Schizzo1" along normal blind 1.2 contours L71 L75 L76 L77 L78 | L69 L81 L82 L83 L84 bodies 7
sketch "Joint Holder 1 Side" plane through (0, -48.4102, 0) normal (0, -1, 0) x (1, 0, 0)
  line L0 (-78.8911, 0) -> (-54.8911, 0)
  line L1 (-54.8911, 0) -> (-54.8911, 5.5)
  line L2 (-54.8911, 5.5) -> (-78.8911, 5.5)
  line L3 (-78.8911, 5.5) -> (-78.8911, 0)
  line L4 (-78.8911, 5.5) -> (-54.8911, 5.5) construction
  line L5 (-54.8911, 5.5) -> (-54.8911, 0) construction
  line L6 (-54.8911, 0) -> (-78.8911, 0) construction
  line L7 (-78.8911, 0) -> (-78.8911, 5.5) construction
  line L8 (-66.8911, 0) -> (-66.8911, 5.5) construction
  line L9 (-78.8911, 6) -> (-54.8911, 6) construction
  line L10 (-66.8911, 5.5) -> (-66.8911, 6) construction
  circle A0 centre (-66.8911, 6) radius 5
  line L11 (-66.8911, 6) -> (-66.8911, 11) construction
  point P0 (-54.8911, 0)
  point P1 (-75.8911, 0)
  dimension "d270" = 6
  dimension "d271" = 10
  constraint horizontal L4
  constraint vertical L5
  constraint horizontal L6
  constraint vertical L7
  constraint coincident L2.end L3.start
  constraint coincident P0 L0.end
  constraint midpoint L6 L8.start
  constraint midpoint L4 L8.end
  constraint perpendicular L8 L9
  constraint midpoint L9 L10.end
  constraint coincident L10.end A0.centre
  constraint coincident A0 L11.end
  constraint perpendicular L9 L11
  constraint collinear L8 L11
  measures "d270" distance of L9 P1
  measures "d271" diameter of A0
extrude "Estrusione64" cut sketch "Joint Holder 1 Side" against normal blind 25 contours L2 A0 picked at (-67.4833, 3.686) bodies 7
sketch "Joint Holder 1 Slot" plane through (0, 0, 5.5) normal (0, 0, 1) x (-1, 0, 0)
  line L0 (71.8661, 48.4102) -> (71.8661, 24.4102)
  line L1 (71.8661, 24.4102) -> (78.8911, 24.4102)
  line L2 (78.8911, 24.4102) -> (78.8911, 48.4102)
  line L3 (78.8911, 48.4102) -> (71.8661, 48.4102)
  line L4 (78.8911, 24.4102) -> (54.8911, 24.4102) construction
  line L5 (54.8911, 24.4102) -> (54.8911, 48.4102) construction
  line L6 (54.8911, 48.4102) -> (78.8911, 48.4102) construction
  line L7 (78.8911, 48.4102) -> (78.8911, 24.4102) construction
  line L8 (78.8911, 36.4102) -> (54.8911, 36.4102) construction
  line L9 (66.8911, 24.4102) -> (66.8911, 48.4102) construction
  line L10 (61.9162, 48.4102) -> (71.8661, 48.4102) construction
  line L11 (71.8661, 48.4102) -> (71.8661, 24.4102) construction
  line L12 (71.8661, 24.4102) -> (61.9162, 24.4102) construction
  line L13 (61.9162, 24.4102) -> (61.9162, 48.4102) construction
  line L14 (61.9162, 48.4102) -> (71.8661, 24.4102) construction
  line L15 (71.8661, 48.4102) -> (61.9162, 24.4102) construction
  line L16 (78.8911, 38.4102) -> (54.8911, 38.4102) construction
  line L17 (62.9162, 48.4102) -> (62.9162, 24.4102) construction
  line L18 (62.9162, 38.4102) -> (61.9162, 38.4102)
  line L19 (61.9162, 38.4102) -> (61.9162, 42.4102)
  line L20 (61.9162, 42.4102) -> (62.9162, 42.4102)
  line L21 (62.9162, 42.4102) -> (62.9162, 38.4102)
  circle A0 centre (75.8911, 38.4102) radius 1.6
  point P0 (54.8911, 48.4102)
  point P1 (66.8911, 36.4102)
  dimension "d274" = 1
  dimension "d277" = 4
  dimension "d294" = 10
  constraint horizontal L4
  constraint vertical L5
  constraint horizontal L6
  constraint vertical L7
  constraint coincident L1.end L2.start
  constraint coincident P0 L5.end
  constraint midpoint L7 L8.start
  constraint midpoint L5 L8.end
  constraint midpoint L4 L9.start
  constraint midpoint L6 L9.end
  constraint horizontal L10
  constraint perpendicular L10 L11
  constraint parallel L10 L12
  constraint parallel L11 L13
  constraint coincident L14 P1
  constraint coincident L15 P1
  constraint midpoint L8 P1
  constraint coincident L0.end L1.start
  constraint coincident L7 L16.start
  constraint coincident L5 L16.end
  constraint perpendicular L5 L16
  constraint coincident L6 L17.start
  constraint perpendicular L4 L17
  constraint coincident L4 L17.end
  constraint horizontal L18
  constraint vertical L19
  constraint horizontal L20
  constraint vertical L21
  constraint coincident L16 L18.start
  constraint coincident L17 L18.start
  constraint collinear L13 L19
  measures "d274" distance of L13 L17
  measures "d277" distance of L18.start L20.end
  measures "d294" distance of L6 L16
revolve "Rivoluzione6" add sketch "Joint Holder 1 Slot" angle 180 about axis through (-66.8911, -24.4102, 5.5) along (0, 1, 0) contours L18 L19 L20 L21 bodies 7
extrude "Estrusione65" add sketch "Schizzo1" along normal blind 10 separate body contours L85 L86 L87 L88 L92 L93 L95 makes body 8
sketch "Schizzo24" plane through (0, -87.8199, 0) normal (0, -1, 0) x (1, 0, 0)
  line L0 (-78.8911, 0) -> (-54.8911, 0)
  line L1 (-54.8911, 0) -> (-54.8911, 10)
  line L2 (-54.8911, 10) -> (-78.8911, 10)
  line L3 (-78.8911, 10) -> (-78.8911, 0)
  line L4 (-78.8911, 10) -> (-54.8911, 10) construction
  line L5 (-54.8911, 10) -> (-54.8911, 0) construction
  line L6 (-54.8911, 0) -> (-78.8911, 0) construction
  line L7 (-78.8911, 0) -> (-78.8911, 10) construction
  line L8 (-66.8911, 10) -> (-66.8911, 0) construction
  circle A0 centre (-66.8911, 10) radius 5
  dimension "d288" = 10
  constraint horizontal L4
  constraint vertical L5
  constraint horizontal L6
  constraint vertical L7
  constraint coincident L2.end L3.start
  constraint coincident L0.end L1.start
  constraint midpoint L4 L8.start
  constraint midpoint L6 L8.end
  constraint coincident L8.start A0.centre
  measures "d288" diameter of A0
extrude "Estrusione66" cut sketch "Schizzo24" against normal blind 25 contours L2 A0 picked at (-65.8928, 7.8335) bodies 8
sketch "Schizzo26" plane through (0, 0, 10) normal (0, 0, 1) x (-1, 0, 0)
  circle A0 centre (75.8911, 77.8199) radius 1.4
  line L0 (71.8911, 87.8199) -> (71.8911, 74.8199)
  line L1 (71.8911, 74.8199) -> (71.8911, 63.8199)
  line L2 (71.8911, 63.8199) -> (78.8911, 63.8199)
  line L3 (78.8911, 63.8199) -> (78.8911, 87.8199)
  line L4 (78.8911, 87.8199) -> (71.8911, 87.8199)
  line L5 (78.8911, 63.8199) -> (54.8911, 63.8199) construction
  line L6 (54.8911, 63.8199) -> (54.8911, 87.8199) construction
  line L7 (54.8911, 87.8199) -> (78.8911, 87.8199) construction
  line L8 (78.8911, 87.8199) -> (78.8911, 63.8199) construction
  line L9 (78.8911, 83.8199) -> (54.8911, 83.8199) construction
  line L10 (78.8911, 77.8199) -> (54.8911, 77.8199) construction
  line L11 (66.8911, 63.8199) -> (66.8911, 87.8199) construction
  line L12 (70.8911, 63.8199) -> (70.8911, 87.8199) construction
  line L13 (71.8911, 77.8199) -> (70.8911, 77.8199)
  line L14 (70.8911, 77.8199) -> (70.8911, 81.8199)
  line L15 (70.8911, 81.8199) -> (71.8911, 81.8199)
  line L16 (71.8911, 81.8199) -> (71.8911, 77.8199)
  line L17 (71.8911, 83.8199) -> (70.8911, 83.8199)
  line L18 (70.8911, 83.8199) -> (70.8911, 87.8199)
  line L19 (70.8911, 87.8199) -> (71.8911, 87.8199)
  line L20 (71.8911, 87.8199) -> (71.8911, 83.8199)
  line L21 (76.8911, 74.8199) -> (78.8911, 74.8199)
  line L22 (78.8911, 74.8199) -> (78.8911, 80.8199)
  line L23 (78.8911, 80.8199) -> (76.8911, 80.8199)
  line L24 (76.8911, 80.8199) -> (76.8911, 74.8199)
  line L25 (76.8911, 74.8199) -> (78.8911, 80.8199) construction
  line L26 (78.8911, 74.8199) -> (76.8911, 80.8199) construction
  line L27 (56.8911, 74.8199) -> (54.8911, 74.8199)
  line L28 (54.8911, 80.8199) -> (56.8911, 80.8199)
  line L29 (56.8911, 80.8199) -> (56.8911, 74.8199)
  line L30 (54.8911, 74.8199) -> (54.8911, 80.8199)
  point P0 (54.8911, 87.8199)
  point P1 (77.8911, 77.8199)
  point P2 (54.8911, 77.8199)
  dimension "d295" = 4
  dimension "d296" = 6
  dimension "d297" = 4
  dimension "d298" = 4
  dimension "d300" = 6
  dimension "d301" = 2
  constraint horizontal L5
  constraint vertical L6
  constraint horizontal L7
  constraint vertical L8
  constraint coincident P0 L6.end
  constraint coincident L2.end L3.start
  constraint coincident L8 L9.start
  constraint coincident L6 L9.end
  constraint perpendicular L8 L9
  constraint coincident L8 L10.start
  constraint coincident L6 P2
  constraint perpendicular L6 L10
  constraint midpoint L5 L11.start
  constraint midpoint L7 L11.end
  constraint coincident L5 L12.start
  constraint coincident L7 L12.end
  constraint perpendicular L7 L12
  constraint horizontal L13
  constraint vertical L14
  constraint horizontal L15
  constraint vertical L16
  constraint coincident L10 L13.start
  constraint coincident L0 L13.start
  constraint horizontal L17
  constraint vertical L18
  constraint horizontal L19
  constraint vertical L20
  constraint coincident L9 L17.start
  constraint coincident L0 L17.start
  constraint horizontal L21
  constraint perpendicular L21 L22
  constraint parallel L21 L23
  constraint parallel L22 L24
  constraint coincident L25 P1
  constraint coincident L26 P1
  constraint coincident L10 P1
  constraint collinear L8 L22
  constraint symmetric L10.start L11 P2
  constraint symmetric L11 L21.start L27.start
  constraint symmetric L11 L21.end L27.end
  constraint symmetric L11 L22.end L28.start
  constraint symmetric L11 L23.end L28.end
  measures "d295" distance of L7 L9
  measures "d296" distance of L9 L10
  measures "d297" distance of L11 L12
  measures "d298" distance of L13.start L15.end
  measures "d300" distance of L21.end L22.end
  measures "d301" distance of L22 L24
extrude "Estrusione67" cut sketch "Schizzo26" against normal blind 1.2 contours A0 L3 L21 L22 L23 L24 | L27 L28 L29 L30 bodies 8
revolve "Rivoluzione5" add sketch "Schizzo26" angle 180 about axis through (-66.8911, -63.8199, 10) along (0, -1, 0) contours L0 L17 L18 L19 L20 | L0 L13 L14 L15 L16 bodies 8
extrude "Estrusione68" add sketch "Schizzo1" along normal blind 140 separate body contours L98 L102 L105 L106 L111 | L98 L102 L103 L106 L110 L111 | L100 L102 L104 L105 L111 | L98 L102 L103 L106 L110 L113 | L100 L102 L103 L104 L111 L112 | L98 L102 L106 L107 L113 L156 L157 L158 | L100 L102 L103 L104 L112 L113 | L100 L102 L104 L107 L113 | L107 L156 L157 L158 L159 | L166 L167 L168 L169 makes body 9
extrude "Estrusione69" add sketch "Schizzo1" along normal blind 16 contours L98 L101 L102 L105 | L100 L101 L102 L105 | L98 L99 L102 L107 L159 | L99 L100 L102 L107 bodies 9
extrude "Estrusione70" cut sketch "Schizzo1" along normal blind 16.5 contours L98 L102 L103 L106 L110 L111 | L98 L102 L103 L106 L110 L113 | L100 L102 L103 L104 L111 L112 | L100 L102 L103 L104 L112 L113 bodies 9
extrude "Estrusione92" cut sketch "Schizzo1" along normal blind 2 contours L107 L156 L157 L158 L159 bodies 9
sketch "Schizzo37" plane through (0, -10.9044, 0) normal (0, 1, 0) x (-1, 0, 0)
  line L0 (261.8139, 0) -> (261.8139, 16.5)
  line L1 (261.8139, 16.5) -> (264.8139, 16.5)
  line L2 (264.8139, 16.5) -> (264.8139, 0)
  line L3 (264.8139, 0) -> (273.3139, 0)
  line L4 (273.3139, 0) -> (273.3139, 16)
  line L5 (273.3139, 16) -> (271.3139, 16)
  line L6 (271.3139, 16) -> (271.3139, 140)
  line L7 (271.3139, 140) -> (255.3139, 140)
  line L8 (255.3139, 140) -> (255.3139, 16)
  line L9 (255.3139, 16) -> (253.3139, 16)
  line L10 (253.3139, 16) -> (253.3139, 0)
  line L11 (253.3139, 0) -> (261.8139, 0)
  line L12 (273.3139, 0) -> (253.3139, 0) construction
  line L13 (253.3139, 0) -> (253.3139, 16) construction
  line L14 (253.3139, 16) -> (273.3139, 16) construction
  line L15 (273.3139, 16) -> (273.3139, 0) construction
  line L16 (273.3139, 8) -> (253.3139, 8) construction
  line L17 (263.3139, 0) -> (263.3139, 16.5) construction
  line L18 (257.8139, 0) -> (257.8139, 16) construction
  line L19 (259.8139, 15.25) -> (255.8139, 15.25)
  line L20 (255.8139, 15.25) -> (255.8139, 0.75)
  line L21 (255.8139, 0.75) -> (259.8139, 0.75)
  line L22 (259.8139, 0.75) -> (259.8139, 15.25)
  line L23 (259.8139, 15.25) -> (255.8139, 0.75) construction
  line L24 (255.8139, 15.25) -> (259.8139, 0.75) construction
  point P0 (257.8139, 8)
  dimension "d406" = 4.5
  dimension "d407" = 4
  dimension "d408" = 14.5
  constraint horizontal L12
  constraint vertical L13
  constraint horizontal L14
  constraint vertical L15
  constraint coincident L3.end L4.start
  constraint coincident L9.end L10.start
  constraint midpoint L15 L16.start
  constraint midpoint L13 L16.end
  constraint midpoint L12 L17.start
  constraint midpoint L1 L17.end
  constraint coincident L11 L18.start
  constraint coincident L14 L18.end
  constraint perpendicular L14 L18
  constraint horizontal L19
  constraint perpendicular L19 L20
  constraint parallel L19 L21
  constraint parallel L20 L22
  constraint coincident L23 P0
  constraint coincident L24 P0
  constraint midpoint L18 P0
  measures "d406" distance of L13 L18
  measures "d407" distance of L20.end L21.end
  measures "d408" distance of L19.end L20.end
extrude "Estrusione94" cut sketch "Schizzo37" against normal blind 5 contours L19 L20 L21 L22 bodies 9
extrude "Estrusione93" cut sketch "Schizzo1" against normal blind 2 from surface at 140 contours L166 L167 L168 L169 bodies 9
sketch "Schizzo33" plane through (0, 0, 140) normal (0, 0, 1) x (-1, 0, 0)
  line L0 (269.8139, 24.9044) -> (265.8139, 24.9044)
  line L1 (265.8139, 24.9044) -> (265.8139, 28.9044)
  line L2 (265.8139, 28.9044) -> (269.8139, 28.9044)
  line L3 (269.8139, 28.9044) -> (269.8139, 24.9044)
  line L4 (255.3139, 10.9044) -> (271.3139, 10.9044)
  line L5 (271.3139, 10.9044) -> (271.3139, 30.9044)
  line L6 (271.3139, 30.9044) -> (255.3139, 30.9044)
  line L7 (255.3139, 30.9044) -> (255.3139, 10.9044)
  line L8 (271.3139, 10.9044) -> (255.3139, 10.9044) construction
  line L9 (255.3139, 10.9044) -> (255.3139, 30.9044) construction
  line L10 (255.3139, 30.9044) -> (271.3139, 30.9044) construction
  line L11 (271.3139, 30.9044) -> (271.3139, 10.9044) construction
  line L12 (269.8139, 24.9044) -> (265.8139, 24.9044) construction
  line L13 (265.8139, 24.9044) -> (265.8139, 28.9044) construction
  line L14 (265.8139, 28.9044) -> (269.8139, 28.9044) construction
  line L15 (269.8139, 28.9044) -> (269.8139, 24.9044) construction
  line L16 (267.8139, 24.9044) -> (269.8139, 24.9044) construction
  line L17 (269.8139, 24.9044) -> (269.8139, 26.9044) construction
  line L18 (269.8139, 26.9044) -> (267.8139, 26.9044) construction
  line L19 (267.8139, 26.9044) -> (267.8139, 24.9044) construction
  constraint horizontal L8
  constraint vertical L9
  constraint horizontal L10
  constraint vertical L11
  constraint coincident L6.end L7.start
  constraint coincident L4.end L5.start
  constraint horizontal L12
  constraint vertical L13
  constraint horizontal L14
  constraint vertical L15
  constraint coincident L1.end L2.start
  constraint coincident L0.start L3.end
  constraint horizontal L16
  constraint vertical L17
  constraint horizontal L18
  constraint vertical L19
  constraint midpoint L15 L17.end
  constraint midpoint L12 L16.start
ref_plane "Piano di lavoro4" through (-257.3139, -10.9044, 0) normal (0.997199, 0, 0.07479) x (0, 1, 0)
sketch "Schizzo36" plane through (-255.8746, 0, -19.1906) normal (0.997199, 0, 0.07479) x (0, 1, 0)
  line L0 (-15.9, 19.2) -> (-27.9, 162.4)
pipe "Tubo2" cut square section size 4 path "Schizzo36" along L0 bodies 9
sketch "Schizzo31" plane through (0, 0, 140) normal (0, 0, 1) x (-1, 0, 0)
  line L0 (255.3139, 10.9044) -> (271.3139, 10.9044)
  line L1 (271.3139, 10.9044) -> (271.3139, 30.9044)
  line L2 (271.3139, 30.9044) -> (255.3139, 30.9044)
  line L3 (255.3139, 30.9044) -> (255.3139, 10.9044)
  line L4 (271.3139, 10.9044) -> (255.3139, 10.9044) construction
  line L5 (255.3139, 10.9044) -> (255.3139, 30.9044) construction
  line L6 (255.3139, 30.9044) -> (271.3139, 30.9044) construction
  line L7 (271.3139, 30.9044) -> (271.3139, 10.9044) construction
  line L8 (271.3139, 20.9044) -> (255.3139, 20.9044) construction
  line L9 (263.3139, 10.9044) -> (263.3139, 30.9044) construction
  line L10 (255.3139, 22.4044) -> (271.3139, 22.4044)
  line L11 (271.3139, 22.4044) -> (271.3139, 19.4044)
  line L12 (271.3139, 19.4044) -> (255.3139, 19.4044)
  line L13 (255.3139, 19.4044) -> (255.3139, 22.4044)
  line L14 (255.3139, 22.4044) -> (271.3139, 19.4044) construction
  line L15 (271.3139, 22.4044) -> (255.3139, 19.4044) construction
  line L16 (269.8195, 25.6741) -> (269.8139, 25.674)
  line L17 (265.8083, 25.6489) -> (265.8083, 29.663)
  line L18 (265.8139, 24.9044) -> (265.8139, 25.649)
  line L19 (269.8139, 25.674) -> (269.8139, 24.9044)
  line L20 (269.8195, 29.6881) -> (269.8195, 25.6741)
  line L21 (265.8083, 29.663) -> (269.8195, 29.6881)
  line L22 (269.8139, 24.9044) -> (265.8139, 24.9044)
  line L23 (265.8139, 25.649) -> (265.8083, 25.6489)
  point P0 (263.3139, 20.9044)
  dimension "d356" = 3
  constraint horizontal L4
  constraint vertical L5
  constraint horizontal L6
  constraint vertical L7
  constraint coincident L2.end L3.start
  constraint coincident L0.end L1.start
  constraint midpoint L7 L8.start
  constraint midpoint L5 L8.end
  constraint midpoint L4 L9.start
  constraint midpoint L2 L9.end
  constraint horizontal L10
  constraint perpendicular L10 L11
  constraint parallel L10 L12
  constraint parallel L11 L13
  constraint coincident L14 P0
  constraint coincident L15 P0
  constraint midpoint L8 P0
  constraint collinear L5 L13
  measures "d356" distance of L10.end L11.end
extrude "Estrusione96" cut sketch "Schizzo31" against normal blind 16.5 contours L1 L3 L10 L11 L12 L13 bodies 9